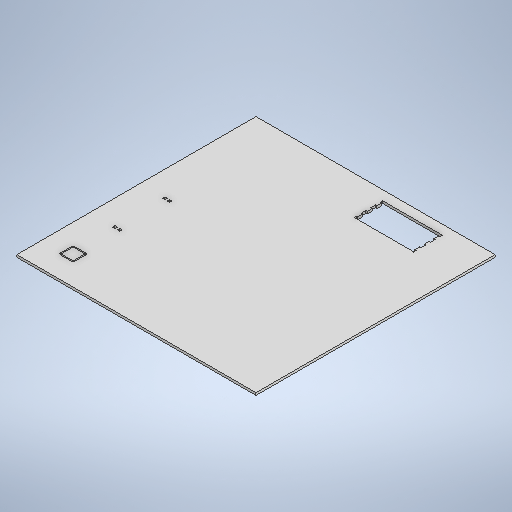
# Autodesk Inventor part: Base
Saved by Autodesk Inventor 2025.3 (Build 293356000, 356)
## iProperties
Created: 2026-04-18
Part Number: Base
Material: Generic
Document SubType Name: Modeling
Designer: kamal
Density: 1 g/cm^3
Appearance: Default
Author: kamal
Autodesk Inventor part; units mm, degrees
ref_plane "YZ Plane" through (0, 0, 0) normal (1, 0, 0) x (0, 1, 0)
ref_plane "XZ Plane" through (0, 0, 0) normal (0, 1, 0) x (-1, 0, 0)
ref_plane "XY Plane" through (0, 0, 0) normal (0, 0, 1) x (1, 0, 0)
sketch "Sketch1" plane through (0, 0, 0) normal (0, 1, 0) x (-1, 0, 0)
  line L0 (-500, 500) -> (500, 500)
  line L1 (500, 500) -> (500, -500)
  line L2 (500, -500) -> (-500, -500)
  line L3 (-500, -500) -> (-500, 500)
  line L4 (-500, 500) -> (500, -500) construction
  line L5 (500, 500) -> (-500, -500) construction
  point P0 (0, 0)
  dimension "d0" = 1000
  dimension "d1" = 1000
  constraints: 12 end point, 2 midpoint, 2 parallel, 1 horizontal, 1 perpendicular
  measures "d0" distance of L1.end L2.end
  measures "d1" distance of L0.end L1.end
extrude "Extrusion1" add sketch "Sketch1" along normal blind 10
sketch "Sketch2" plane through (0, 10, 0) normal (0, 1, 0) x (1, 0, 0)
  line L0 (-400, -200) -> (-370, -200)
  line L1 (-370, -200) -> (-370, -190)
  line L2 (-370, -190) -> (-400, -190)
  line L3 (-400, -190) -> (-400, -200)
  line L4 (-500, 500) -> (-500, -500) projected
  line L5 (-500, -500) -> (500, -500) projected
  line L6 (-390, -190) -> (-390, -200)
  line L7 (-380, -190) -> (-380, -200)
  point P0 (0, 0)
  point P1 (-400, -195)
  point P2 (-390, -195)
  point P3 (-380, -195)
  dimension "d5" = 30
  dimension "d6" = 10
  dimension "d7" = 100
  dimension "d8" = 300
  dimension "d9" = 10
  dimension "d10" = 10
  constraints: 12 end point, 4 point on line, 3 midpoint, 3 perpendicular, 2 parallel, 1 horizontal
  measures "d5" distance of L2.end L1.end
  measures "d6" distance of L1.end L0.end
  measures "d7" distance from line of point (-400, -195) L4
  measures "d8" distance between parallel lines of L5 L0
  measures "d9" distance of point (-400, -195) point (-390, -195)
  measures "d10" distance from line of L1 point (-380, -195)
extrude "Extrusion2" cut sketch "Sketch2" against normal blind 10 contours L3 L2 L6 L0 | L7 L2 L1 L0
sketch "Sketch3" plane through (0, 10, 0) normal (0, 1, 0) x (1, 0, 0)
  line L0 (-400, -190) -> (-390, -190) projected
  line L1 (-400, -200) -> (-400, -190) projected
  line L2 (-390, -190) -> (-390, -200) projected
  line L3 (-390, -200) -> (-400, -200) projected
  line L4 (-380, -200) -> (-380, -190) projected
  line L5 (-380, -190) -> (-370, -190) projected
  line L6 (-370, -190) -> (-370, -200) projected
  line L7 (-370, -200) -> (-380, -200) projected
  line L8 (-400, 8.6) -> (-370, 8.6)
  line L9 (-370, 8.6) -> (-370, 18.6)
  line L10 (-370, 18.6) -> (-400, 18.6)
  line L11 (-400, 18.6) -> (-400, 8.6)
  line L12 (-380, 8.6) -> (-380, 18.6)
  line L13 (-390, 8.6) -> (-390, 18.6)
  point P0 (0, 0)
  point P1 (-380, 13.6)
  point P2 (-375, -190)
  dimension "d13" = 30
  dimension "d14" = 10
  dimension "d15" = 10
  dimension "d16" = 10
  dimension "d17" = 198.6
  dimension "d18" = 10
  constraints: 12 end point, 4 point on line, 3 perpendicular, 2 midpoint, 2 parallel, 1 horizontal
  measures "d13" distance of L10.end L9.end
  measures "d14" distance of L9.end L8.end
  measures "d15" distance from line of point (-380, 13.6) L13
  measures "d16" distance between parallel lines of L13 L11
  measures "d17" distance from line of point (-375, -190) L8
  measures "d18" distance between parallel lines of L6 L12
extrude "Extrusion3" cut sketch "Sketch3" against normal blind 10 contours L11 L10 L13 L8 | L12 L10 L9 L8
sketch "Sketch4" plane through (0, 10, 0) normal (0, 1, 0) x (1, 0, 0)
  line L0 (-405, -400) -> (-365, -400)
  line L1 (-365, -400) -> (-365, -360)
  line L2 (-365, -360) -> (-405, -360)
  line L3 (-405, -360) -> (-405, -400)
  line L4 (-405, -400) -> (-365, -360) construction
  line L5 (-365, -400) -> (-405, -360) construction
  line L6 (-500, 500) -> (-500, -500) projected
  line L7 (-500, -500) -> (500, -500) projected
  line L8 (-410, -355) -> (-360, -355)
  line L9 (-360, -355) -> (-360, -405)
  line L10 (-360, -405) -> (-410, -405)
  line L11 (-410, -405) -> (-410, -355)
  line L12 (-355, -350) -> (-415, -350)
  line L13 (-415, -350) -> (-415, -410)
  line L14 (-415, -410) -> (-355, -410)
  line L15 (-355, -410) -> (-355, -350)
  line L16 (-410, -355) -> (-415, -355)
  line L17 (-410, -355) -> (-410, -350)
  line L18 (-360, -355) -> (-360, -350)
  line L19 (-360, -355) -> (-355, -355)
  line L20 (-410, -405) -> (-410, -410)
  line L21 (-410, -405) -> (-415, -405)
  line L22 (-360, -405) -> (-360, -410)
  line L23 (-360, -405) -> (-355, -405)
  point P0 (0, 0)
  point P1 (-385, -380)
  point P2 (-405, -380)
  dimension "d21" = 40
  dimension "d22" = 40
  dimension "d23" = 95
  dimension "d24" = 100
  dimension "d25" = 5
  dimension "d26" = 5
  constraints: 44 end point, 12 point on line, 6 parallel, 6 perpendicular, 3 midpoint, 2 horizontal, 6 other
  measures "d21" distance of L2.end L1.end
  measures "d22" distance of L1.end L0.end
  measures "d23" distance from line of L6 point (-405, -380)
  measures "d24" distance between parallel lines of L7 L0
  measures "d25" distance between parallel lines of L2 L8
  measures "d26" distance between parallel lines of L8 L12
extrude "Extrusion4" cut sketch "Sketch4" against normal blind 10 contours L17 L12 L18 L8 | L11 L21 L13 L16 | L19 L15 L23 L9 | L10 L22 L14 L20
sketch "Sketch5" plane through (0, 10, 0) normal (0, 1, 0) x (1, 0, 0)
  line L0 (120, 340) -> (120, 460)
  circle A0 centre (200, 400) radius 50
  line L1 (120, 340) -> (270, 340)
  line L2 (270, 460) -> (120, 460)
  line L3 (120, 460) -> (120, 450)
  line L4 (120, 450) -> (126, 450)
  line L5 (126, 450) -> (126, 430)
  line L6 (126, 430) -> (120, 430)
  line L7 (120, 430) -> (120, 410)
  line L8 (120, 410) -> (126, 410)
  line L9 (126, 410) -> (126, 390)
  line L10 (126, 390) -> (120, 390)
  line L11 (120, 390) -> (120, 370)
  line L12 (120, 370) -> (126, 370)
  line L13 (126, 370) -> (126, 350)
  line L14 (126, 350) -> (120, 350)
  line L15 (120, 460) -> (70, 460)
  line L16 (70, 460) -> (70, 450)
  line L17 (70, 450) -> (76, 450)
  line L18 (76, 450) -> (76, 430)
  line L19 (76, 430) -> (70, 430)
  line L20 (70, 430) -> (70, 410)
  line L21 (70, 410) -> (76, 410)
  line L22 (76, 410) -> (76, 390)
  line L23 (76, 390) -> (70, 390)
  line L24 (70, 390) -> (70, 370)
  line L25 (70, 370) -> (76, 370)
  line L26 (76, 370) -> (76, 350)
  line L27 (76, 350) -> (70, 350)
  line L28 (70, 350) -> (70, 340)
  line L29 (70, 340) -> (120, 340)
  line L30 (272.052, 455.4405) -> (266.0681, 455)
  line L31 (266.0681, 455) -> (267.5363, 435.054)
  line L32 (270, 460) -> (320, 460)
  line L33 (320, 460) -> (320, 450)
  line L34 (320, 450) -> (314, 450)
  line L35 (314, 450) -> (314, 430)
  line L36 (314, 430) -> (320, 430)
  line L37 (320, 430) -> (320, 410)
  line L38 (320, 410) -> (314, 410)
  line L39 (314, 410) -> (314, 390)
  line L40 (314, 390) -> (320, 390)
  line L41 (320, 390) -> (320, 370)
  line L42 (320, 370) -> (314, 370)
  line L43 (314, 370) -> (314, 350)
  line L44 (314, 350) -> (320, 350)
  line L45 (320, 350) -> (320, 340)
  line L46 (320, 340) -> (270, 340)
  line L47 (270, 460) -> (270, 340)
  line L48 (267.5363, 435.054) -> (270, 435.054)
  line L49 (270, 435.054) -> (270, 430.054)
  line L50 (270, 430.054) -> (266.0681, 430.054)
  line L51 (266.0681, 430.054) -> (266.0681, 410.054)
  line L52 (266.0681, 410.054) -> (270, 410.054)
  line L53 (120, 460) -> (120, 466)
  line L54 (272.0681, 465) -> (270, 460)
  line L55 (120, 466) -> (130, 466)
  line L56 (130, 466) -> (130, 460)
  line L57 (130, 460) -> (150, 460)
  line L58 (150, 460) -> (150, 466)
  line L59 (150, 466) -> (170, 466)
  line L60 (170, 466) -> (170, 460)
  line L61 (170, 460) -> (190, 460)
  line L62 (190, 460) -> (190, 466)
  line L63 (190, 466) -> (210, 466)
  line L64 (210, 466) -> (210, 460)
  line L65 (210, 460) -> (230, 460)
  line L66 (230, 460) -> (230, 466)
  line L67 (230, 466) -> (250, 466)
  line L68 (250, 466) -> (250, 460)
  line L69 (250, 460) -> (260, 460)
  line L70 (260, 460) -> (260, 465)
  line L71 (260, 465) -> (272.0681, 465)
  line L72 (500, 500) -> (-500, 500) projected
  line L73 (500, -500) -> (500, 500) projected
  point P0 (0, 0)
  dimension "d29" = 100
  dimension "d30" = 120
  dimension "d31" = 150
  dimension "d32" = 80
  dimension "d33" = 60
  dimension "d34" = 10
  dimension "d35" = 6
  dimension "d36" = 20
  dimension "d37" = 20
  dimension "d38" = 20
  dimension "d39" = 20
  dimension "d40" = 20
  dimension "d41" = 50
  dimension "d42" = 10
  dimension "d43" = 6
  dimension "d44" = 5
  dimension "d45" = 6
  dimension "d46" = 50
  dimension "d47" = 6
  dimension "d48" = 5
  dimension "d49" = 20
  dimension "d50" = 20
  dimension "d51" = 6
  dimension "d52" = 10
  dimension "d53" = 20
  dimension "d54" = 20
  dimension "d55" = 20
  dimension "d56" = 20
  dimension "d57" = 20
  dimension "d58" = 20
  dimension "d59" = 10
  dimension "d60" = 100
  dimension "d61" = 300
  constraints: 142 end point, 39 point on line, 31 perpendicular, 8 vertical, 6 horizontal, 1 centre point, 1 parallel, 11 other
  measures "d29" diameter of A0
  measures "d30" distance of L0.start L0.end
  measures "d31" distance of L32.start L0.end
  measures "d32" distance from line of L0 A0.centre
  measures "d34" distance of L0.end L4.start
  measures "d35" distance of L4.start L4.end
  measures "d36" distance of L4.end L6.start
  measures "d37" distance of L6.end L8.start
  measures "d38" distance of L8.end L9.end
  measures "d39" distance of L10.end L11.end
  measures "d40" distance of L12.end L13.end
  measures "d41" distance of L0.end L15.end
  measures "d42" distance of L15.end L17.start
  measures "d43" distance of L17.start L18.start
  measures "d44" distance of L32.start L30.start
  measures "d45" distance of L30.start L30.end
  measures "d46" distance of L32.start L32.end
  measures "d47" distance of L34.start L34.end
  measures "d48" distance between parallel lines of L50 L48
  measures "d49" distance of L50.end L52.start
  measures "d50" distance of L30.end L31.end
  measures "d51" distance of L0.end L55.start
  measures "d52" distance of L55.start L55.end
  measures "d53" distance of L57.start L58.start
  measures "d54" distance of L58.end L60.start
  measures "d55" distance of L61.start L61.end
  measures "d56" distance of L62.end L64.start
  measures "d57" distance of L65.start L66.start
  measures "d58" distance of L66.end L68.start
  measures "d59" distance of L68.end L70.start
  measures "d60" distance from line of L72 A0.centre
  measures "d61" distance from line of L73 A0.centre
extrude "Extrusion5" cut sketch "Sketch5" against normal blind 80 contours L29 L28 L27 L26 L25 L24 L23 L22 L21 L20 L19 L18 L17 L16 L15 L0 | L0 L14 L13 L12 L10 L9 L8 L6 L5 L4 L2 L47 L30 L31 L48 L50 L51 L52 L1 | L0 L12 L13 L14 | L47 L32 L33 L34 L35 L36 L37 L38 L39 L40 L41 L42 L43 L44 L45 L46 | L52 L51 L50 L47 | L0 L8 L9 L10 | L48 L31 L30 L47 | L0 L4 L5 L6 | A0
equation "\"d62\" = d32"
body "Solid1"
